Autodesk Fusion 360 part; units mm, degrees
(part 7 of 8)
equation "d1212 = ( BaseX + LeftRun + FaucetGap + ( RightRun + ModuleGap ) / 2 ) + ( ( ( RightRun - ModuleGap ) / 2 ) / 2 - 8 mm )"
equation "d1213 = ( BaseY ) + ( ( Depth ) - Wall - DeckClearance - 4 mm )"
equation "d1216 = DeckThick"
equation "d1220 = ( BaseX + LeftRun + FaucetGap + ( RightRun + ModuleGap ) / 2 ) + ( ( 11 mm ) - FootSize / 2 )"
equation "d1221 = ( BaseY ) + ( ( 11 mm ) - FootSize / 2 )"
equation "d1222 = FootSize"
equation "d1223 = FootSize"
equation "d1224 = FootHeight"
equation "d1226 = FootHeight"
equation "d1228 = ( BaseX + LeftRun + FaucetGap + ( RightRun + ModuleGap ) / 2 ) + ( ( 11 mm ) - PegSize / 2 )"
equation "d1229 = ( BaseY ) + ( ( 11 mm ) - PegSize / 2 )"
equation "d1230 = PegSize"
equation "d1231 = PegSize"
equation "d1232 = PegHeight"
equation "d1236 = ( BaseX + LeftRun + FaucetGap + ( RightRun + ModuleGap ) / 2 ) + ( ( 11 mm ) - FootSize / 2 )"
equation "d1237 = ( BaseY ) + ( ( ( Depth ) - 11 mm ) - FootSize / 2 )"
equation "d1238 = FootSize"
equation "d1239 = FootSize"
equation "d1240 = FootHeight"
equation "d1242 = FootHeight"
equation "d1244 = ( BaseX + LeftRun + FaucetGap + ( RightRun + ModuleGap ) / 2 ) + ( ( 11 mm ) - PegSize / 2 )"
equation "d1245 = ( BaseY ) + ( ( ( Depth ) - 11 mm ) - PegSize / 2 )"
equation "d1246 = PegSize"
equation "d1247 = PegSize"
equation "d1248 = PegHeight"
equation "d1252 = ( BaseX + LeftRun + FaucetGap + ( RightRun + ModuleGap ) / 2 ) + ( ( ( ( RightRun - ModuleGap ) / 2 ) - 11 mm ) - FootSize / 2 )"
equation "d1253 = ( BaseY ) + ( ( 11 mm ) - FootSize / 2 )"
equation "d1254 = FootSize"
equation "d1255 = FootSize"
equation "d1256 = FootHeight"
equation "d1258 = FootHeight"
equation "d1260 = ( BaseX + LeftRun + FaucetGap + ( RightRun + ModuleGap ) / 2 ) + ( ( ( ( RightRun - ModuleGap ) / 2 ) - 11 mm ) - PegSize / 2 )"
equation "d1261 = ( BaseY ) + ( ( 11 mm ) - PegSize / 2 )"
equation "d1262 = PegSize"
equation "d1263 = PegSize"
equation "d1264 = PegHeight"
equation "d1268 = ( BaseX + LeftRun + FaucetGap + ( RightRun + ModuleGap ) / 2 ) + ( ( ( ( RightRun - ModuleGap ) / 2 ) - 11 mm ) - FootSize / 2 )"
equation "d1269 = ( BaseY ) + ( ( ( Depth ) - 11 mm ) - FootSize / 2 )"
equation "d1270 = FootSize"
equation "d1271 = FootSize"
equation "d1272 = FootHeight"
equation "d1274 = FootHeight"
equation "d1276 = ( BaseX + LeftRun + FaucetGap + ( RightRun + ModuleGap ) / 2 ) + ( ( ( ( RightRun - ModuleGap ) / 2 ) - 11 mm ) - PegSize / 2 )"
equation "d1277 = ( BaseY ) + ( ( ( Depth ) - 11 mm ) - PegSize / 2 )"
equation "d1278 = PegSize"
equation "d1279 = PegSize"
equation "d1280 = PegHeight"
equation "d1282 = FootHeight"
equation "d1284 = ( BaseX ) + ( 0 mm )"
equation "d1285 = ( BaseY + Depth + ModuleGap ) + ( ( LeftReach ) - ( ( 0 mm ) + ( LeftReach ) ) )"
equation "d1286 = LeftSideDepth"
equation "d1287 = LeftReach"
equation "d1288 = PanHeight"
equation "d1292 = ( BaseY + Depth + ModuleGap ) + ( ( LeftReach ) - ( Wall ) )"
equation "d1294 = ( ( BaseX ) + ( Wall ) )"
equation "d1295 = -( -( ( FootHeight ) + FloorMin + DrainExtension * tan(DrainSlope) + ( ( LeftSideDepth ) - ( Wall ) ) * tan(DrainSlope) ) )"
equation "d1296 = ( ( BaseX ) + ( ( LeftSideDepth ) - Wall ) )"
equation "d1297 = -( -( ( FootHeight ) + FloorMin + DrainExtension * tan(DrainSlope) + ( ( LeftSideDepth ) - ( ( LeftSideDepth ) - Wall ) ) * tan(DrainSlope) ) )"
equation "d1298 = -( -( ( FootHeight ) + PanHeight + 1 mm ) )"
equation "d1299 = -( -( -( ( LeftReach ) - 2 * Wall ) ) )"
equation "d1301 = ( BaseY + Depth + ModuleGap ) + ( ( LeftReach ) - ( ( LeftReach / 2 ) - DrainWidth / 2 - Wall ) )"
equation "d1303 = ( ( BaseX ) + ( ( LeftSideDepth ) - Wall ) )"
equation "d1304 = -( -( FootHeight ) )"
equation "d1305 = ( ( BaseX ) + ( ( LeftSideDepth ) + DrainExtension ) )"
equation "d1306 = -( -( ( FootHeight ) + FloorMin + DrainExtension * tan(DrainSlope) + ( ( LeftSideDepth ) - ( ( LeftSideDepth ) + DrainExtension ) ) * tan(DrainSlope) ) )"
equation "d1307 = -( -( ( FootHeight ) + FloorMin + DrainExtension * tan(DrainSlope) + ( ( LeftSideDepth ) - ( ( LeftSideDepth ) - Wall ) ) * tan(DrainSlope) ) )"
equation "d1308 = -( DrainWidth + 2 * Wall )"
equation "d1310 = ( BaseY + Depth + ModuleGap ) + ( ( LeftReach ) - ( ( LeftReach / 2 ) - DrainWidth / 2 - Wall ) )"
equation "d1312 = ( ( BaseX ) + ( ( LeftSideDepth ) - Wall ) )"
equation "d1313 = -( -( FootHeight ) )"
equation "d1314 = ( ( BaseX ) + ( ( LeftSideDepth ) + DrainExtension ) )"
equation "d1315 = -( -( ( ( FootHeight ) + FloorMin + DrainExtension * tan(DrainSlope) + ( ( LeftSideDepth ) - ( ( LeftSideDepth ) + DrainExtension ) ) * tan(DrainSlope) ) + ( 6 mm ) ) )"
equation "d1316 = -( -( ( ( FootHeight ) + FloorMin + DrainExtension * tan(DrainSlope) + ( ( LeftSideDepth ) - ( ( LeftSideDepth ) - Wall ) ) * tan(DrainSlope) ) + ( 6 mm ) ) )"
equation "d1317 = -( Wall )"
equation "d1319 = ( BaseY + Depth + ModuleGap ) + ( ( LeftReach ) - ( ( LeftReach / 2 ) + DrainWidth / 2 ) )"
equation "d1321 = ( ( BaseX ) + ( ( LeftSideDepth ) - Wall ) )"
equation "d1322 = -( -( FootHeight ) )"
equation "d1323 = ( ( BaseX ) + ( ( LeftSideDepth ) + DrainExtension ) )"
equation "d1324 = -( -( ( ( FootHeight ) + FloorMin + DrainExtension * tan(DrainSlope) + ( ( LeftSideDepth ) - ( ( LeftSideDepth ) + DrainExtension ) ) * tan(DrainSlope) ) + ( 6 mm ) ) )"
equation "d1325 = -( -( ( ( FootHeight ) + FloorMin + DrainExtension * tan(DrainSlope) + ( ( LeftSideDepth ) - ( ( LeftSideDepth ) - Wall ) ) * tan(DrainSlope) ) + ( 6 mm ) ) )"
equation "d1326 = -( Wall )"
equation "d1328 = ( BaseY + Depth + ModuleGap ) + ( ( LeftReach ) - ( ( LeftReach / 2 ) - DrainWidth / 2 ) )"
equation "d1330 = ( ( BaseX ) + ( ( LeftSideDepth ) - Wall ) )"
equation "d1331 = -( -( ( FootHeight ) + FloorMin + DrainExtension * tan(DrainSlope) + ( ( LeftSideDepth ) - ( ( LeftSideDepth ) - Wall ) ) * tan(DrainSlope) ) )"
equation "d1332 = ( ( BaseX ) + ( ( LeftSideDepth ) + DrainExtension ) )"
equation "d1333 = -( -( ( FootHeight ) + FloorMin + DrainExtension * tan(DrainSlope) + ( ( LeftSideDepth ) - ( ( LeftSideDepth ) + DrainExtension ) ) * tan(DrainSlope) ) )"
equation "d1334 = -( -( ( FootHeight ) + PanHeight + 1 mm ) )"
equation "d1335 = -( -( -( DrainWidth ) ) )"
equation "d1337 = FootHeight"
equation "d1339 = ( BaseX ) + ( Wall )"
equation "d1340 = ( BaseY + Depth + ModuleGap ) + ( ( LeftReach ) - ( ( Wall ) + ( 12 mm ) ) )"
equation "d1343 = PanHeight - DeckThick"
equation "d1345 = FootHeight"
equation "d1347 = ( BaseX ) + ( ( LeftSideDepth ) - Wall - 12 mm )"
equation "d1348 = ( BaseY + Depth + ModuleGap ) + ( ( LeftReach ) - ( ( Wall ) + ( 12 mm ) ) )"
equation "d1351 = PanHeight - DeckThick"
equation "d1353 = FootHeight"
equation "d1355 = ( BaseX ) + ( Wall )"
equation "d1356 = ( BaseY + Depth + ModuleGap ) + ( ( LeftReach ) - ( ( ( LeftReach ) - Wall - 12 mm ) + ( 12 mm ) ) )"
equation "d1359 = PanHeight - DeckThick"
equation "d1361 = FootHeight"
equation "d1363 = ( BaseX ) + ( ( LeftSideDepth ) - Wall - 12 mm )"
equation "d1364 = ( BaseY + Depth + ModuleGap ) + ( ( LeftReach ) - ( ( ( LeftReach ) - Wall - 12 mm ) + ( 12 mm ) ) )"
equation "d1367 = PanHeight - DeckThick"
equation "d1369 = ( BaseY + Depth + ModuleGap ) + ( ( LeftReach ) - ( ( LeftReach / 2 ) - DrainWidth / 2 - Wall ) )"
equation "d1371 = ( ( BaseX ) + ( ( LeftSideDepth ) + DrainExtension - 2 mm ) )"
equation "d1372 = -( -( ( FootHeight ) - ( 0.2 mm ) ) )"
equation "d1373 = ( ( BaseX ) + ( ( ( LeftSideDepth ) + DrainExtension - 2 mm ) + ( 1 mm ) ) )"
equation "d1374 = -( -( ( FootHeight ) + ( 0.6 mm ) ) )"
equation "d1375 = -( -( -( DrainWidth + 2 * Wall ) ) )"
equation "d1377 = FootHeight"
equation "d1379 = ( BaseX ) + ( ( 11 mm ) - PegSize / 2 - FitClearance )"
equation "d1380 = ( BaseY + Depth + ModuleGap ) + ( ( LeftReach ) - ( ( ( 11 mm ) - PegSize / 2 - FitClearance ) + ( PegSize + 2 * FitClearance ) ) )"
equation "d1381 = PegSize + 2 * FitClearance"
equation "d1382 = PegSize + 2 * FitClearance"
equation "d1383 = PegHeight + 0.3 mm"
equation "d1385 = FootHeight"
equation "d1387 = ( BaseX ) + ( ( ( LeftSideDepth ) - 11 mm ) - PegSize / 2 - FitClearance )"
equation "d1388 = ( BaseY + Depth + ModuleGap ) + ( ( LeftReach ) - ( ( ( 11 mm ) - PegSize / 2 - FitClearance ) + ( PegSize + 2 * FitClearance ) ) )"
equation "d1389 = PegSize + 2 * FitClearance"
equation "d1390 = PegSize + 2 * FitClearance"
equation "d1391 = PegHeight + 0.3 mm"
equation "d1393 = FootHeight"
equation "d1395 = ( BaseX ) + ( ( 11 mm ) - PegSize / 2 - FitClearance )"
equation "d1396 = ( BaseY + Depth + ModuleGap ) + ( ( LeftReach ) - ( ( ( ( LeftReach ) - 11 mm ) - PegSize / 2 - FitClearance ) + ( PegSize + 2 * FitClearance ) ) )"
equation "d1397 = PegSize + 2 * FitClearance"
equation "d1398 = PegSize + 2 * FitClearance"
equation "d1399 = PegHeight + 0.3 mm"
equation "d1401 = FootHeight"
equation "d1403 = ( BaseX ) + ( ( ( LeftSideDepth ) - 11 mm ) - PegSize / 2 - FitClearance )"
equation "d1404 = ( BaseY + Depth + ModuleGap ) + ( ( LeftReach ) - ( ( ( ( LeftReach ) - 11 mm ) - PegSize / 2 - FitClearance ) + ( PegSize + 2 * FitClearance ) ) )"
equation "d1405 = PegSize + 2 * FitClearance"
equation "d1406 = PegSize + 2 * FitClearance"
equation "d1407 = PegHeight + 0.3 mm"
equation "d1409 = ( FootHeight ) + PanHeight - DeckThick"
equation "d1411 = ( BaseX ) + ( Wall + DeckClearance )"
equation "d1412 = ( BaseY + Depth + ModuleGap ) + ( ( LeftReach ) - ( ( Wall + DeckClearance ) + ( ( LeftReach ) - 2 * ( Wall + DeckClearance ) ) ) )"
equation "d1413 = ( LeftSideDepth ) - 2 * ( Wall + DeckClearance )"
equation "d1414 = ( LeftReach ) - 2 * ( Wall + DeckClearance )"
equation "d1415 = DeckThick"
equation "d1417 = ( FootHeight ) + PanHeight - DeckThick"
equation "d1419 = ( BaseX ) + ( Wall + DeckClearance + RimBorder )"
equation "d1420 = ( BaseY + Depth + ModuleGap ) + ( ( LeftReach ) - ( ( ( ( ( LeftReach ) - ( 14 * SlotPitch + SlotWidth ) ) / 2 ) + ( 0 * SlotPitch ) ) + ( SlotWidth ) ) )"
equation "d1421 = ( LeftSideDepth ) - 2 * ( Wall + DeckClearance + RimBorder )"
equation "d1422 = SlotWidth"
equation "d1423 = DeckThick"
equation "d1425 = ( FootHeight ) + PanHeight - DeckThick"
equation "d1427 = ( BaseX ) + ( Wall + DeckClearance + RimBorder )"
equation "d1428 = ( BaseY + Depth + ModuleGap ) + ( ( LeftReach ) - ( ( ( ( ( LeftReach ) - ( 14 * SlotPitch + SlotWidth ) ) / 2 ) + ( 1 * SlotPitch ) ) + ( SlotWidth ) ) )"
equation "d1429 = ( LeftSideDepth ) - 2 * ( Wall + DeckClearance + RimBorder )"
equation "d1430 = SlotWidth"
equation "d1431 = DeckThick"
equation "d1433 = ( FootHeight ) + PanHeight - DeckThick"
equation "d1435 = ( BaseX ) + ( Wall + DeckClearance + RimBorder )"
equation "d1436 = ( BaseY + Depth + ModuleGap ) + ( ( LeftReach ) - ( ( ( ( ( LeftReach ) - ( 14 * SlotPitch + SlotWidth ) ) / 2 ) + ( 2 * SlotPitch ) ) + ( SlotWidth ) ) )"
equation "d1437 = ( LeftSideDepth ) - 2 * ( Wall + DeckClearance + RimBorder )"
equation "d1438 = SlotWidth"
equation "d1439 = DeckThick"
equation "d1441 = ( FootHeight ) + PanHeight - DeckThick"
equation "d1443 = ( BaseX ) + ( Wall + DeckClearance + RimBorder )"
equation "d1444 = ( BaseY + Depth + ModuleGap ) + ( ( LeftReach ) - ( ( ( ( ( LeftReach ) - ( 14 * SlotPitch + SlotWidth ) ) / 2 ) + ( 3 * SlotPitch ) ) + ( SlotWidth ) ) )"
equation "d1445 = ( LeftSideDepth ) - 2 * ( Wall + DeckClearance + RimBorder )"
equation "d1446 = SlotWidth"
equation "d1447 = DeckThick"
equation "d1449 = ( FootHeight ) + PanHeight - DeckThick"
equation "d1451 = ( BaseX ) + ( Wall + DeckClearance + RimBorder )"
equation "d1452 = ( BaseY + Depth + ModuleGap ) + ( ( LeftReach ) - ( ( ( ( ( LeftReach ) - ( 14 * SlotPitch + SlotWidth ) ) / 2 ) + ( 4 * SlotPitch ) ) + ( SlotWidth ) ) )"
equation "d1453 = ( LeftSideDepth ) - 2 * ( Wall + DeckClearance + RimBorder )"
equation "d1454 = SlotWidth"
equation "d1455 = DeckThick"
equation "d1457 = ( FootHeight ) + PanHeight - DeckThick"
equation "d1459 = ( BaseX ) + ( Wall + DeckClearance + RimBorder )"
equation "d1460 = ( BaseY + Depth + ModuleGap ) + ( ( LeftReach ) - ( ( ( ( ( LeftReach ) - ( 14 * SlotPitch + SlotWidth ) ) / 2 ) + ( 5 * SlotPitch ) ) + ( SlotWidth ) ) )"
equation "d1461 = ( LeftSideDepth ) - 2 * ( Wall + DeckClearance + RimBorder )"
equation "d1462 = SlotWidth"
equation "d1463 = DeckThick"
equation "d1465 = ( FootHeight ) + PanHeight - DeckThick"
equation "d1467 = ( BaseX ) + ( Wall + DeckClearance + RimBorder )"
equation "d1468 = ( BaseY + Depth + ModuleGap ) + ( ( LeftReach ) - ( ( ( ( ( LeftReach ) - ( 14 * SlotPitch + SlotWidth ) ) / 2 ) + ( 6 * SlotPitch ) ) + ( SlotWidth ) ) )"
equation "d1469 = ( LeftSideDepth ) - 2 * ( Wall + DeckClearance + RimBorder )"
equation "d1470 = SlotWidth"
equation "d1471 = DeckThick"
equation "d1473 = ( FootHeight ) + PanHeight - DeckThick"
equation "d1475 = ( BaseX ) + ( Wall + DeckClearance + RimBorder )"
equation "d1476 = ( BaseY + Depth + ModuleGap ) + ( ( LeftReach ) - ( ( ( ( ( LeftReach ) - ( 14 * SlotPitch + SlotWidth ) ) / 2 ) + ( 7 * SlotPitch ) ) + ( SlotWidth ) ) )"
equation "d1477 = ( LeftSideDepth ) - 2 * ( Wall + DeckClearance + RimBorder )"
equation "d1478 = SlotWidth"
equation "d1479 = DeckThick"
equation "d1481 = ( FootHeight ) + PanHeight - DeckThick"
equation "d1483 = ( BaseX ) + ( Wall + DeckClearance + RimBorder )"
equation "d1484 = ( BaseY + Depth + ModuleGap ) + ( ( LeftReach ) - ( ( ( ( ( LeftReach ) - ( 14 * SlotPitch + SlotWidth ) ) / 2 ) + ( 8 * SlotPitch ) ) + ( SlotWidth ) ) )"
equation "d1485 = ( LeftSideDepth ) - 2 * ( Wall + DeckClearance + RimBorder )"
equation "d1486 = SlotWidth"
equation "d1487 = DeckThick"
equation "d1489 = ( FootHeight ) + PanHeight - DeckThick"
equation "d1491 = ( BaseX ) + ( Wall + DeckClearance + RimBorder )"
equation "d1492 = ( BaseY + Depth + ModuleGap ) + ( ( LeftReach ) - ( ( ( ( ( LeftReach ) - ( 14 * SlotPitch + SlotWidth ) ) / 2 ) + ( 9 * SlotPitch ) ) + ( SlotWidth ) ) )"
equation "d1493 = ( LeftSideDepth ) - 2 * ( Wall + DeckClearance + RimBorder )"
equation "d1494 = SlotWidth"
equation "d1495 = DeckThick"
equation "d1497 = ( FootHeight ) + PanHeight - DeckThick"
equation "d1499 = ( BaseX ) + ( Wall + DeckClearance + RimBorder )"
equation "d1500 = ( BaseY + Depth + ModuleGap ) + ( ( LeftReach ) - ( ( ( ( ( LeftReach ) - ( 14 * SlotPitch + SlotWidth ) ) / 2 ) + ( 10 * SlotPitch ) ) + ( SlotWidth ) ) )"
equation "d1501 = ( LeftSideDepth ) - 2 * ( Wall + DeckClearance + RimBorder )"
equation "d1502 = SlotWidth"
equation "d1503 = DeckThick"
equation "d1505 = ( FootHeight ) + PanHeight - DeckThick"
equation "d1507 = ( BaseX ) + ( Wall + DeckClearance + RimBorder )"
equation "d1508 = ( BaseY + Depth + ModuleGap ) + ( ( LeftReach ) - ( ( ( ( ( LeftReach ) - ( 14 * SlotPitch + SlotWidth ) ) / 2 ) + ( 11 * SlotPitch ) ) + ( SlotWidth ) ) )"
equation "d1509 = ( LeftSideDepth ) - 2 * ( Wall + DeckClearance + RimBorder )"
equation "d1510 = SlotWidth"
equation "d1511 = DeckThick"
equation "d1513 = ( FootHeight ) + PanHeight - DeckThick"
equation "d1515 = ( BaseX ) + ( Wall + DeckClearance + RimBorder )"
equation "d1516 = ( BaseY + Depth + ModuleGap ) + ( ( LeftReach ) - ( ( ( ( ( LeftReach ) - ( 14 * SlotPitch + SlotWidth ) ) / 2 ) + ( 12 * SlotPitch ) ) + ( SlotWidth ) ) )"
equation "d1517 = ( LeftSideDepth ) - 2 * ( Wall + DeckClearance + RimBorder )"
equation "d1518 = SlotWidth"
equation "d1519 = DeckThick"
equation "d1521 = ( FootHeight ) + PanHeight - DeckThick"
equation "d1523 = ( BaseX ) + ( Wall + DeckClearance + RimBorder )"
equation "d1524 = ( BaseY + Depth + ModuleGap ) + ( ( LeftReach ) - ( ( ( ( ( LeftReach ) - ( 14 * SlotPitch + SlotWidth ) ) / 2 ) + ( 13 * SlotPitch ) ) + ( SlotWidth ) ) )"
equation "d1525 = ( LeftSideDepth ) - 2 * ( Wall + DeckClearance + RimBorder )"
equation "d1526 = SlotWidth"
equation "d1527 = DeckThick"
equation "d1529 = ( FootHeight ) + PanHeight - DeckThick"
equation "d1531 = ( BaseX ) + ( Wall + DeckClearance + RimBorder )"
equation "d1532 = ( BaseY + Depth + ModuleGap ) + ( ( LeftReach ) - ( ( ( ( ( LeftReach ) - ( 14 * SlotPitch + SlotWidth ) ) / 2 ) + ( 14 * SlotPitch ) ) + ( SlotWidth ) ) )"
equation "d1533 = ( LeftSideDepth ) - 2 * ( Wall + DeckClearance + RimBorder )"
equation "d1534 = SlotWidth"
equation "d1535 = DeckThick"
equation "d1537 = ( FootHeight ) + PanHeight - DeckThick"
equation "d1539 = ( BaseX ) + ( ( LeftSideDepth ) - Wall - DeckClearance - 4 mm )"
equation "d1540 = ( BaseY + Depth + ModuleGap ) + ( ( LeftReach ) - ( ( ( LeftReach ) / 2 - 8 mm ) + ( 16 mm ) ) )"
equation "d1543 = DeckThick"
equation "d1547 = ( BaseX ) + ( ( 11 mm ) - FootSize / 2 )"
equation "d1548 = ( BaseY + Depth + ModuleGap ) + ( ( LeftReach ) - ( ( ( 11 mm ) - FootSize / 2 ) + ( FootSize ) ) )"
equation "d1549 = FootSize"
equation "d1550 = FootSize"
equation "d1551 = FootHeight"
equation "d1553 = FootHeight"
equation "d1555 = ( BaseX ) + ( ( 11 mm ) - PegSize / 2 )"
equation "d1556 = ( BaseY + Depth + ModuleGap ) + ( ( LeftReach ) - ( ( ( 11 mm ) - PegSize / 2 ) + ( PegSize ) ) )"
equation "d1557 = PegSize"
equation "d1558 = PegSize"
equation "d1559 = PegHeight"
equation "d1563 = ( BaseX ) + ( ( ( LeftSideDepth ) - 11 mm ) - FootSize / 2 )"
equation "d1564 = ( BaseY + Depth + ModuleGap ) + ( ( LeftReach ) - ( ( ( 11 mm ) - FootSize / 2 ) + ( FootSize ) ) )"
equation "d1565 = FootSize"
equation "d1566 = FootSize"
equation "d1567 = FootHeight"
equation "d1569 = FootHeight"
equation "d1571 = ( BaseX ) + ( ( ( LeftSideDepth ) - 11 mm ) - PegSize / 2 )"
equation "d1572 = ( BaseY + Depth + ModuleGap ) + ( ( LeftReach ) - ( ( ( 11 mm ) - PegSize / 2 ) + ( PegSize ) ) )"
equation "d1573 = PegSize"
equation "d1574 = PegSize"
equation "d1575 = PegHeight"
equation "d1579 = ( BaseX ) + ( ( 11 mm ) - FootSize / 2 )"
equation "d1580 = ( BaseY + Depth + ModuleGap ) + ( ( LeftReach ) - ( ( ( ( LeftReach ) - 11 mm ) - FootSize / 2 ) + ( FootSize ) ) )"
equation "d1581 = FootSize"
equation "d1582 = FootSize"
equation "d1583 = FootHeight"
equation "d1585 = FootHeight"
equation "d1587 = ( BaseX ) + ( ( 11 mm ) - PegSize / 2 )"
equation "d1588 = ( BaseY + Depth + ModuleGap ) + ( ( LeftReach ) - ( ( ( ( LeftReach ) - 11 mm ) - PegSize / 2 ) + ( PegSize ) ) )"
equation "d1589 = PegSize"
equation "d1590 = PegSize"
equation "d1591 = PegHeight"
equation "d1595 = ( BaseX ) + ( ( ( LeftSideDepth ) - 11 mm ) - FootSize / 2 )"
equation "d1596 = ( BaseY + Depth + ModuleGap ) + ( ( LeftReach ) - ( ( ( ( LeftReach ) - 11 mm ) - FootSize / 2 ) + ( FootSize ) ) )"
equation "d1597 = FootSize"
equation "d1598 = FootSize"
equation "d1599 = FootHeight"
equation "d1601 = FootHeight"
equation "d1603 = ( BaseX ) + ( ( ( LeftSideDepth ) - 11 mm ) - PegSize / 2 )"
equation "d1604 = ( BaseY + Depth + ModuleGap ) + ( ( LeftReach ) - ( ( ( ( LeftReach ) - 11 mm ) - PegSize / 2 ) + ( PegSize ) ) )"
equation "d1605 = PegSize"
equation "d1606 = PegSize"
equation "d1607 = PegHeight"
equation "d1609 = FootHeight"
equation "d1611 = ( BaseX + LeftRun + FaucetGap + RightRun - RightSideDepth ) + ( ( RightSideDepth ) - ( ( 0 mm ) + ( RightSideDepth ) ) )"
equation "d1612 = ( BaseY + Depth + ModuleGap ) + ( 0 mm )"
equation "d1613 = RightSideDepth"
equation "d1614 = RightReach"
equation "d1615 = PanHeight"
equation "d1619 = ( BaseY + Depth + ModuleGap ) + ( Wall )"
equation "d1621 = ( ( BaseX + LeftRun + FaucetGap + RightRun - RightSideDepth ) + ( ( RightSideDepth ) - ( Wall ) ) )"
equation "d1622 = -( -( ( FootHeight ) + FloorMin + DrainExtension * tan(DrainSlope) + ( ( RightSideDepth ) - ( Wall ) ) * tan(DrainSlope) ) )"
equation "d1623 = ( ( BaseX + LeftRun + FaucetGap + RightRun - RightSideDepth ) + ( ( RightSideDepth ) - ( ( RightSideDepth ) - Wall ) ) )"
equation "d1624 = -( -( ( FootHeight ) + FloorMin + DrainExtension * tan(DrainSlope) + ( ( RightSideDepth ) - ( ( RightSideDepth ) - Wall ) ) * tan(DrainSlope) ) )"
equation "d1625 = -( -( ( FootHeight ) + PanHeight + 1 mm ) )"
equation "d1626 = ( RightReach ) - 2 * Wall"
equation "d1628 = ( BaseY + Depth + ModuleGap ) + ( ( RightReach / 2 ) - DrainWidth / 2 - Wall )"
equation "d1630 = ( ( BaseX + LeftRun + FaucetGap + RightRun - RightSideDepth ) + ( ( RightSideDepth ) - ( ( RightSideDepth ) - Wall ) ) )"
equation "d1631 = -( -( FootHeight ) )"
equation "d1632 = ( ( BaseX + LeftRun + FaucetGap + RightRun - RightSideDepth ) + ( ( RightSideDepth ) - ( ( RightSideDepth ) + DrainExtension ) ) )"
equation "d1633 = -( -( ( FootHeight ) + FloorMin + DrainExtension * tan(DrainSlope) + ( ( RightSideDepth ) - ( ( RightSideDepth ) + DrainExtension ) ) * tan(DrainSlope) ) )"
equation "d1634 = -( -( ( FootHeight ) + FloorMin + DrainExtension * tan(DrainSlope) + ( ( RightSideDepth ) - ( ( RightSideDepth ) - Wall ) ) * tan(DrainSlope) ) )"
equation "d1635 = DrainWidth + 2 * Wall"
equation "d1637 = ( BaseY + Depth + ModuleGap ) + ( ( RightReach / 2 ) - DrainWidth / 2 - Wall )"
equation "d1639 = ( ( BaseX + LeftRun + FaucetGap + RightRun - RightSideDepth ) + ( ( RightSideDepth ) - ( ( RightSideDepth ) - Wall ) ) )"
equation "d1640 = -( -( FootHeight ) )"
equation "d1641 = ( ( BaseX + LeftRun + FaucetGap + RightRun - RightSideDepth ) + ( ( RightSideDepth ) - ( ( RightSideDepth ) + DrainExtension ) ) )"
equation "d1642 = -( -( ( ( FootHeight ) + FloorMin + DrainExtension * tan(DrainSlope) + ( ( RightSideDepth ) - ( ( RightSideDepth ) + DrainExtension ) ) * tan(DrainSlope) ) + ( 6 mm ) ) )"
equation "d1643 = -( -( ( ( FootHeight ) + FloorMin + DrainExtension * tan(DrainSlope) + ( ( RightSideDepth ) - ( ( RightSideDepth ) - Wall ) ) * tan(DrainSlope) ) + ( 6 mm ) ) )"
equation "d1644 = Wall"
equation "d1646 = ( BaseY + Depth + ModuleGap ) + ( ( RightReach / 2 ) + DrainWidth / 2 )"
equation "d1648 = ( ( BaseX + LeftRun + FaucetGap + RightRun - RightSideDepth ) + ( ( RightSideDepth ) - ( ( RightSideDepth ) - Wall ) ) )"
equation "d1649 = -( -( FootHeight ) )"
equation "d1650 = ( ( BaseX + LeftRun + FaucetGap + RightRun - RightSideDepth ) + ( ( RightSideDepth ) - ( ( RightSideDepth ) + DrainExtension ) ) )"
equation "d1651 = -( -( ( ( FootHeight ) + FloorMin + DrainExtension * tan(DrainSlope) + ( ( RightSideDepth ) - ( ( RightSideDepth ) + DrainExtension ) ) * tan(DrainSlope) ) + ( 6 mm ) ) )"
equation "d1652 = -( -( ( ( FootHeight ) + FloorMin + DrainExtension * tan(DrainSlope) + ( ( RightSideDepth ) - ( ( RightSideDepth ) - Wall ) ) * tan(DrainSlope) ) + ( 6 mm ) ) )"
equation "d1653 = Wall"
equation "d1655 = ( BaseY + Depth + ModuleGap ) + ( ( RightReach / 2 ) - DrainWidth / 2 )"
equation "d1657 = ( ( BaseX + LeftRun + FaucetGap + RightRun - RightSideDepth ) + ( ( RightSideDepth ) - ( ( RightSideDepth ) - Wall ) ) )"
equation "d1658 = -( -( ( FootHeight ) + FloorMin + DrainExtension * tan(DrainSlope) + ( ( RightSideDepth ) - ( ( RightSideDepth ) - Wall ) ) * tan(DrainSlope) ) )"
equation "d1659 = ( ( BaseX + LeftRun + FaucetGap + RightRun - RightSideDepth ) + ( ( RightSideDepth ) - ( ( RightSideDepth ) + DrainExtension ) ) )"
equation "d1660 = -( -( ( FootHeight ) + FloorMin + DrainExtension * tan(DrainSlope) + ( ( RightSideDepth ) - ( ( RightSideDepth ) + DrainExtension ) ) * tan(DrainSlope) ) )"
equation "d1661 = -( -( ( FootHeight ) + PanHeight + 1 mm ) )"
equation "d1662 = DrainWidth"
equation "d1664 = FootHeight"
equation "d1666 = ( BaseX + LeftRun + FaucetGap + RightRun - RightSideDepth ) + ( ( RightSideDepth ) - ( ( Wall ) + ( 12 mm ) ) )"
equation "d1667 = ( BaseY + Depth + ModuleGap ) + ( Wall )"
equation "d1670 = PanHeight - DeckThick"
equation "d1672 = FootHeight"
equation "d1674 = ( BaseX + LeftRun + FaucetGap + RightRun - RightSideDepth ) + ( ( RightSideDepth ) - ( ( ( RightSideDepth ) - Wall - 12 mm ) + ( 12 mm ) ) )"
equation "d1675 = ( BaseY + Depth + ModuleGap ) + ( Wall )"
equation "d1678 = PanHeight - DeckThick"
equation "d1680 = FootHeight"
equation "d1682 = ( BaseX + LeftRun + FaucetGap + RightRun - RightSideDepth ) + ( ( RightSideDepth ) - ( ( Wall ) + ( 12 mm ) ) )"
equation "d1683 = ( BaseY + Depth + ModuleGap ) + ( ( RightReach ) - Wall - 12 mm )"
equation "d1686 = PanHeight - DeckThick"
equation "d1688 = FootHeight"
equation "d1690 = ( BaseX + LeftRun + FaucetGap + RightRun - RightSideDepth ) + ( ( RightSideDepth ) - ( ( ( RightSideDepth ) - Wall - 12 mm ) + ( 12 mm ) ) )"
equation "d1691 = ( BaseY + Depth + ModuleGap ) + ( ( RightReach ) - Wall - 12 mm )"
equation "d1694 = PanHeight - DeckThick"
equation "d1696 = ( BaseY + Depth + ModuleGap ) + ( ( RightReach / 2 ) - DrainWidth / 2 - Wall )"
equation "d1698 = ( ( BaseX + LeftRun + FaucetGap + RightRun - RightSideDepth ) + ( ( RightSideDepth ) - ( ( RightSideDepth ) + DrainExtension - 2 mm ) ) )"
equation "d1699 = -( -( ( FootHeight ) - ( 0.2 mm ) ) )"
equation "d1700 = ( ( BaseX + LeftRun + FaucetGap + RightRun - RightSideDepth ) + ( ( RightSideDepth ) - ( ( ( RightSideDepth ) + DrainExtension - 2 mm ) + ( 1 mm ) ) ) )"
equation "d1701 = -( -( ( FootHeight ) + ( 0.6 mm ) ) )"
equation "d1702 = DrainWidth + 2 * Wall"
equation "d1704 = FootHeight"
equation "d1706 = ( BaseX + LeftRun + FaucetGap + RightRun - RightSideDepth ) + ( ( RightSideDepth ) - ( ( ( 11 mm ) - PegSize / 2 - FitClearance ) + ( PegSize + 2 * FitClearance ) ) )"
equation "d1707 = ( BaseY + Depth + ModuleGap ) + ( ( 11 mm ) - PegSize / 2 - FitClearance )"
equation "d1708 = PegSize + 2 * FitClearance"
equation "d1709 = PegSize + 2 * FitClearance"
equation "d1710 = PegHeight + 0.3 mm"
equation "d1712 = FootHeight"
equation "d1714 = ( BaseX + LeftRun + FaucetGap + RightRun - RightSideDepth ) + ( ( RightSideDepth ) - ( ( ( ( RightSideDepth ) - 11 mm ) - PegSize / 2 - FitClearance ) + ( PegSize + 2 * FitClearance ) ) )"
equation "d1715 = ( BaseY + Depth + ModuleGap ) + ( ( 11 mm ) - PegSize / 2 - FitClearance )"
equation "d1716 = PegSize + 2 * FitClearance"
equation "d1717 = PegSize + 2 * FitClearance"
equation "d1718 = PegHeight + 0.3 mm"
equation "d1720 = FootHeight"
equation "d1722 = ( BaseX + LeftRun + FaucetGap + RightRun - RightSideDepth ) + ( ( RightSideDepth ) - ( ( ( 11 mm ) - PegSize / 2 - FitClearance ) + ( PegSize + 2 * FitClearance ) ) )"
equation "d1723 = ( BaseY + Depth + ModuleGap ) + ( ( ( RightReach ) - 11 mm ) - PegSize / 2 - FitClearance )"
equation "d1724 = PegSize + 2 * FitClearance"
equation "d1725 = PegSize + 2 * FitClearance"
equation "d1726 = PegHeight + 0.3 mm"
equation "d1728 = FootHeight"
equation "d1730 = ( BaseX + LeftRun + FaucetGap + RightRun - RightSideDepth ) + ( ( RightSideDepth ) - ( ( ( ( RightSideDepth ) - 11 mm ) - PegSize / 2 - FitClearance ) + ( PegSize + 2 * FitClearance ) ) )"
equation "d1731 = ( BaseY + Depth + ModuleGap ) + ( ( ( RightReach ) - 11 mm ) - PegSize / 2 - FitClearance )"
equation "d1732 = PegSize + 2 * FitClearance"
equation "d1733 = PegSize + 2 * FitClearance"
equation "d1734 = PegHeight + 0.3 mm"
equation "d1736 = ( FootHeight ) + PanHeight - DeckThick"
equation "d1738 = ( BaseX + LeftRun + FaucetGap + RightRun - RightSideDepth ) + ( ( RightSideDepth ) - ( ( Wall + DeckClearance ) + ( ( RightSideDepth ) - 2 * ( Wall + DeckClearance ) ) ) )"
equation "d1739 = ( BaseY + Depth + ModuleGap ) + ( Wall + DeckClearance )"
equation "d1740 = ( RightSideDepth ) - 2 * ( Wall + DeckClearance )"
equation "d1741 = ( RightReach ) - 2 * ( Wall + DeckClearance )"
equation "d1742 = DeckThick"
equation "d1744 = ( FootHeight ) + PanHeight - DeckThick"
equation "d1746 = ( BaseX + LeftRun + FaucetGap + RightRun - RightSideDepth ) + ( ( RightSideDepth ) - ( ( Wall + DeckClearance + RimBorder ) + ( ( RightSideDepth ) - 2 * ( Wall + DeckClearance + RimBorder ) ) ) )"
equation "d1747 = ( BaseY + Depth + ModuleGap ) + ( ( ( ( RightReach ) - ( 14 * SlotPitch + SlotWidth ) ) / 2 ) + ( 0 * SlotPitch ) )"
equation "d1748 = ( RightSideDepth ) - 2 * ( Wall + DeckClearance + RimBorder )"
equation "d1749 = SlotWidth"
equation "d1750 = DeckThick"
equation "d1752 = ( FootHeight ) + PanHeight - DeckThick"
equation "d1754 = ( BaseX + LeftRun + FaucetGap + RightRun - RightSideDepth ) + ( ( RightSideDepth ) - ( ( Wall + DeckClearance + RimBorder ) + ( ( RightSideDepth ) - 2 * ( Wall + DeckClearance + RimBorder ) ) ) )"
equation "d1755 = ( BaseY + Depth + ModuleGap ) + ( ( ( ( RightReach ) - ( 14 * SlotPitch + SlotWidth ) ) / 2 ) + ( 1 * SlotPitch ) )"
equation "d1756 = ( RightSideDepth ) - 2 * ( Wall + DeckClearance + RimBorder )"
equation "d1757 = SlotWidth"
equation "d1758 = DeckThick"
equation "d1760 = ( FootHeight ) + PanHeight - DeckThick"
equation "d1762 = ( BaseX + LeftRun + FaucetGap + RightRun - RightSideDepth ) + ( ( RightSideDepth ) - ( ( Wall + DeckClearance + RimBorder ) + ( ( RightSideDepth ) - 2 * ( Wall + DeckClearance + RimBorder ) ) ) )"
equation "d1763 = ( BaseY + Depth + ModuleGap ) + ( ( ( ( RightReach ) - ( 14 * SlotPitch + SlotWidth ) ) / 2 ) + ( 2 * SlotPitch ) )"
equation "d1764 = ( RightSideDepth ) - 2 * ( Wall + DeckClearance + RimBorder )"
equation "d1765 = SlotWidth"
equation "d1766 = DeckThick"
equation "d1768 = ( FootHeight ) + PanHeight - DeckThick"
equation "d1770 = ( BaseX + LeftRun + FaucetGap + RightRun - RightSideDepth ) + ( ( RightSideDepth ) - ( ( Wall + DeckClearance + RimBorder ) + ( ( RightSideDepth ) - 2 * ( Wall + DeckClearance + RimBorder ) ) ) )"
equation "d1771 = ( BaseY + Depth + ModuleGap ) + ( ( ( ( RightReach ) - ( 14 * SlotPitch + SlotWidth ) ) / 2 ) + ( 3 * SlotPitch ) )"
equation "d1772 = ( RightSideDepth ) - 2 * ( Wall + DeckClearance + RimBorder )"
equation "d1773 = SlotWidth"
equation "d1774 = DeckThick"
equation "d1776 = ( FootHeight ) + PanHeight - DeckThick"
equation "d1778 = ( BaseX + LeftRun + FaucetGap + RightRun - RightSideDepth ) + ( ( RightSideDepth ) - ( ( Wall + DeckClearance + RimBorder ) + ( ( RightSideDepth ) - 2 * ( Wall + DeckClearance + RimBorder ) ) ) )"
equation "d1779 = ( BaseY + Depth + ModuleGap ) + ( ( ( ( RightReach ) - ( 14 * SlotPitch + SlotWidth ) ) / 2 ) + ( 4 * SlotPitch ) )"
equation "d1780 = ( RightSideDepth ) - 2 * ( Wall + DeckClearance + RimBorder )"
equation "d1781 = SlotWidth"
equation "d1782 = DeckThick"
equation "d1784 = ( FootHeight ) + PanHeight - DeckThick"
equation "d1786 = ( BaseX + LeftRun + FaucetGap + RightRun - RightSideDepth ) + ( ( RightSideDepth ) - ( ( Wall + DeckClearance + RimBorder ) + ( ( RightSideDepth ) - 2 * ( Wall + DeckClearance + RimBorder ) ) ) )"
equation "d1787 = ( BaseY + Depth + ModuleGap ) + ( ( ( ( RightReach ) - ( 14 * SlotPitch + SlotWidth ) ) / 2 ) + ( 5 * SlotPitch ) )"
equation "d1788 = ( RightSideDepth ) - 2 * ( Wall + DeckClearance + RimBorder )"
equation "d1789 = SlotWidth"
equation "d1790 = DeckThick"
equation "d1792 = ( FootHeight ) + PanHeight - DeckThick"
equation "d1794 = ( BaseX + LeftRun + FaucetGap + RightRun - RightSideDepth ) + ( ( RightSideDepth ) - ( ( Wall + DeckClearance + RimBorder ) + ( ( RightSideDepth ) - 2 * ( Wall + DeckClearance + RimBorder ) ) ) )"
equation "d1795 = ( BaseY + Depth + ModuleGap ) + ( ( ( ( RightReach ) - ( 14 * SlotPitch + SlotWidth ) ) / 2 ) + ( 6 * SlotPitch ) )"
equation "d1796 = ( RightSideDepth ) - 2 * ( Wall + DeckClearance + RimBorder )"
equation "d1797 = SlotWidth"
equation "d1798 = DeckThick"
equation "d1800 = ( FootHeight ) + PanHeight - DeckThick"
equation "d1802 = ( BaseX + LeftRun + FaucetGap + RightRun - RightSideDepth ) + ( ( RightSideDepth ) - ( ( Wall + DeckClearance + RimBorder ) + ( ( RightSideDepth ) - 2 * ( Wall + DeckClearance + RimBorder ) ) ) )"
equation "d1803 = ( BaseY + Depth + ModuleGap ) + ( ( ( ( RightReach ) - ( 14 * SlotPitch + SlotWidth ) ) / 2 ) + ( 7 * SlotPitch ) )"
equation "d1804 = ( RightSideDepth ) - 2 * ( Wall + DeckClearance + RimBorder )"
equation "d1805 = SlotWidth"
equation "d1806 = DeckThick"
equation "d1808 = ( FootHeight ) + PanHeight - DeckThick"
equation "d1810 = ( BaseX + LeftRun + FaucetGap + RightRun - RightSideDepth ) + ( ( RightSideDepth ) - ( ( Wall + DeckClearance + RimBorder ) + ( ( RightSideDepth ) - 2 * ( Wall + DeckClearance + RimBorder ) ) ) )"
equation "d1811 = ( BaseY + Depth + ModuleGap ) + ( ( ( ( RightReach ) - ( 14 * SlotPitch + SlotWidth ) ) / 2 ) + ( 8 * SlotPitch ) )"
equation "d1812 = ( RightSideDepth ) - 2 * ( Wall + DeckClearance + RimBorder )"
equation "d1813 = SlotWidth"
equation "d1814 = DeckThick"
equation "d1816 = ( FootHeight ) + PanHeight - DeckThick"
equation "d1818 = ( BaseX + LeftRun + FaucetGap + RightRun - RightSideDepth ) + ( ( RightSideDepth ) - ( ( Wall + DeckClearance + RimBorder ) + ( ( RightSideDepth ) - 2 * ( Wall + DeckClearance + RimBorder ) ) ) )"
equation "d1819 = ( BaseY + Depth + ModuleGap ) + ( ( ( ( RightReach ) - ( 14 * SlotPitch + SlotWidth ) ) / 2 ) + ( 9 * SlotPitch ) )"
equation "d1820 = ( RightSideDepth ) - 2 * ( Wall + DeckClearance + RimBorder )"
equation "d1821 = SlotWidth"
equation "d1822 = DeckThick"
equation "d1824 = ( FootHeight ) + PanHeight - DeckThick"
equation "d1826 = ( BaseX + LeftRun + FaucetGap + RightRun - RightSideDepth ) + ( ( RightSideDepth ) - ( ( Wall + DeckClearance + RimBorder ) + ( ( RightSideDepth ) - 2 * ( Wall + DeckClearance + RimBorder ) ) ) )"
equation "d1827 = ( BaseY + Depth + ModuleGap ) + ( ( ( ( RightReach ) - ( 14 * SlotPitch + SlotWidth ) ) / 2 ) + ( 10 * SlotPitch ) )"
equation "d1828 = ( RightSideDepth ) - 2 * ( Wall + DeckClearance + RimBorder )"
equation "d1829 = SlotWidth"
equation "d1830 = DeckThick"
equation "d1832 = ( FootHeight ) + PanHeight - DeckThick"
equation "d1834 = ( BaseX + LeftRun + FaucetGap + RightRun - RightSideDepth ) + ( ( RightSideDepth ) - ( ( Wall + DeckClearance + RimBorder ) + ( ( RightSideDepth ) - 2 * ( Wall + DeckClearance + RimBorder ) ) ) )"
equation "d1835 = ( BaseY + Depth + ModuleGap ) + ( ( ( ( RightReach ) - ( 14 * SlotPitch + SlotWidth ) ) / 2 ) + ( 11 * SlotPitch ) )"
equation "d1836 = ( RightSideDepth ) - 2 * ( Wall + DeckClearance + RimBorder )"
equation "d1837 = SlotWidth"
equation "d1838 = DeckThick"
equation "d1840 = ( FootHeight ) + PanHeight - DeckThick"
equation "d1842 = ( BaseX + LeftRun + FaucetGap + RightRun - RightSideDepth ) + ( ( RightSideDepth ) - ( ( Wall + DeckClearance + RimBorder ) + ( ( RightSideDepth ) - 2 * ( Wall + DeckClearance + RimBorder ) ) ) )"
equation "d1843 = ( BaseY + Depth + ModuleGap ) + ( ( ( ( RightReach ) - ( 14 * SlotPitch + SlotWidth ) ) / 2 ) + ( 12 * SlotPitch ) )"
equation "d1844 = ( RightSideDepth ) - 2 * ( Wall + DeckClearance + RimBorder )"
equation "d1845 = SlotWidth"
equation "d1846 = DeckThick"
equation "d1848 = ( FootHeight ) + PanHeight - DeckThick"
equation "d1850 = ( BaseX + LeftRun + FaucetGap + RightRun - RightSideDepth ) + ( ( RightSideDepth ) - ( ( Wall + DeckClearance + RimBorder ) + ( ( RightSideDepth ) - 2 * ( Wall + DeckClearance + RimBorder ) ) ) )"
equation "d1851 = ( BaseY + Depth + ModuleGap ) + ( ( ( ( RightReach ) - ( 14 * SlotPitch + SlotWidth ) ) / 2 ) + ( 13 * SlotPitch ) )"
equation "d1852 = ( RightSideDepth ) - 2 * ( Wall + DeckClearance + RimBorder )"
equation "d1853 = SlotWidth"
equation "d1854 = DeckThick"
equation "d1856 = ( FootHeight ) + PanHeight - DeckThick"
equation "d1858 = ( BaseX + LeftRun + FaucetGap + RightRun - RightSideDepth ) + ( ( RightSideDepth ) - ( ( Wall + DeckClearance + RimBorder ) + ( ( RightSideDepth ) - 2 * ( Wall + DeckClearance + RimBorder ) ) ) )"
equation "d1859 = ( BaseY + Depth + ModuleGap ) + ( ( ( ( RightReach ) - ( 14 * SlotPitch + SlotWidth ) ) / 2 ) + ( 14 * SlotPitch ) )"
equation "d1860 = ( RightSideDepth ) - 2 * ( Wall + DeckClearance + RimBorder )"
equation "d1861 = SlotWidth"
equation "d1862 = DeckThick"
equation "d1864 = ( FootHeight ) + PanHeight - DeckThick"
equation "d1866 = ( BaseX + LeftRun + FaucetGap + RightRun - RightSideDepth ) + ( ( RightSideDepth ) - ( ( ( RightSideDepth ) - Wall - DeckClearance - 4 mm ) + ( 5 mm ) ) )"
equation "d1867 = ( BaseY + Depth + ModuleGap ) + ( ( RightReach ) / 2 - 8 mm )"
equation "d1870 = DeckThick"
equation "d1874 = ( BaseX + LeftRun + FaucetGap + RightRun - RightSideDepth ) + ( ( RightSideDepth ) - ( ( ( 11 mm ) - FootSize / 2 ) + ( FootSize ) ) )"
equation "d1875 = ( BaseY + Depth + ModuleGap ) + ( ( 11 mm ) - FootSize / 2 )"
equation "d1876 = FootSize"
equation "d1877 = FootSize"
equation "d1878 = FootHeight"
equation "d1880 = FootHeight"
equation "d1882 = ( BaseX + LeftRun + FaucetGap + RightRun - RightSideDepth ) + ( ( RightSideDepth ) - ( ( ( 11 mm ) - PegSize / 2 ) + ( PegSize ) ) )"
equation "d1883 = ( BaseY + Depth + ModuleGap ) + ( ( 11 mm ) - PegSize / 2 )"
equation "d1884 = PegSize"
equation "d1885 = PegSize"
equation "d1886 = PegHeight"
equation "d1890 = ( BaseX + LeftRun + FaucetGap + RightRun - RightSideDepth ) + ( ( RightSideDepth ) - ( ( ( ( RightSideDepth ) - 11 mm ) - FootSize / 2 ) + ( FootSize ) ) )"
equation "d1891 = ( BaseY + Depth + ModuleGap ) + ( ( 11 mm ) - FootSize / 2 )"
equation "d1892 = FootSize"
equation "d1893 = FootSize"
equation "d1894 = FootHeight"
equation "d1896 = FootHeight"
equation "d1898 = ( BaseX + LeftRun + FaucetGap + RightRun - RightSideDepth ) + ( ( RightSideDepth ) - ( ( ( ( RightSideDepth ) - 11 mm ) - PegSize / 2 ) + ( PegSize ) ) )"
equation "d1899 = ( BaseY + Depth + ModuleGap ) + ( ( 11 mm ) - PegSize / 2 )"
equation "d1900 = PegSize"
equation "d1901 = PegSize"
equation "d1902 = PegHeight"
equation "d1906 = ( BaseX + LeftRun + FaucetGap + RightRun - RightSideDepth ) + ( ( RightSideDepth ) - ( ( ( 11 mm ) - FootSize / 2 ) + ( FootSize ) ) )"
equation "d1907 = ( BaseY + Depth + ModuleGap ) + ( ( ( RightReach ) - 11 mm ) - FootSize / 2 )"
equation "d1908 = FootSize"
equation "d1909 = FootSize"
equation "d1910 = FootHeight"
equation "d1912 = FootHeight"
equation "d1914 = ( BaseX + LeftRun + FaucetGap + RightRun - RightSideDepth ) + ( ( RightSideDepth ) - ( ( ( 11 mm ) - PegSize / 2 ) + ( PegSize ) ) )"
equation "d1915 = ( BaseY + Depth + ModuleGap ) + ( ( ( RightReach ) - 11 mm ) - PegSize / 2 )"
equation "d1916 = PegSize"
equation "d1917 = PegSize"
equation "d1918 = PegHeight"
equation "d1922 = ( BaseX + LeftRun + FaucetGap + RightRun - RightSideDepth ) + ( ( RightSideDepth ) - ( ( ( ( RightSideDepth ) - 11 mm ) - FootSize / 2 ) + ( FootSize ) ) )"
equation "d1923 = ( BaseY + Depth + ModuleGap ) + ( ( ( RightReach ) - 11 mm ) - FootSize / 2 )"
equation "d1924 = FootSize"
equation "d1925 = FootSize"
equation "d1926 = FootHeight"
equation "d1928 = FootHeight"
equation "d1930 = ( BaseX + LeftRun + FaucetGap + RightRun - RightSideDepth ) + ( ( RightSideDepth ) - ( ( ( ( RightSideDepth ) - 11 mm ) - PegSize / 2 ) + ( PegSize ) ) )"
equation "d1931 = ( BaseY + Depth + ModuleGap ) + ( ( ( RightReach ) - 11 mm ) - PegSize / 2 )"
equation "d1932 = PegSize"
equation "d1933 = PegSize"
equation "d1934 = PegHeight"
equation "d1936 = UpperDeckHeight - PanHeight"
equation "d1938 = ( BaseX ) + ( 0 mm )"
equation "d1939 = ( BaseY ) + ( 0 mm )"
equation "d1940 = TowerWidth"
equation "d1941 = Depth"
equation "d1942 = PanHeight"
equation "d1946 = ( BaseX ) + ( Wall )"
equation "d1948 = -( -( ( UpperDeckHeight - PanHeight ) + FloorMin + DrainExtension * tan(DrainSlope) + ( ( Depth ) - ( Wall ) ) * tan(DrainSlope) ) )"
equation "d1949 = ( ( BaseY ) + ( Wall ) )"
equation "d1950 = -( -( ( UpperDeckHeight - PanHeight ) + FloorMin + DrainExtension * tan(DrainSlope) + ( ( Depth ) - ( ( Depth ) - Wall ) ) * tan(DrainSlope) ) )"
equation "d1951 = ( ( BaseY ) + ( ( Depth ) - Wall ) )"
equation "d1952 = -( -( ( UpperDeckHeight - PanHeight ) + PanHeight + 1 mm ) )"
equation "d1953 = ( TowerWidth ) - 2 * Wall"
equation "d1955 = ( BaseX ) + ( ( TowerWidth - 35 mm ) - DrainWidth / 2 - Wall )"
equation "d1957 = -( -( UpperDeckHeight - PanHeight ) )"
equation "d1958 = ( ( BaseY ) + ( ( Depth ) - Wall ) )"
equation "d1959 = ( ( BaseY ) + ( ( Depth ) + DrainExtension ) )"
equation "d1960 = -( -( ( UpperDeckHeight - PanHeight ) + FloorMin + DrainExtension * tan(DrainSlope) + ( ( Depth ) - ( ( Depth ) + DrainExtension ) ) * tan(DrainSlope) ) )"
equation "d1961 = -( -( ( UpperDeckHeight - PanHeight ) + FloorMin + DrainExtension * tan(DrainSlope) + ( ( Depth ) - ( ( Depth ) - Wall ) ) * tan(DrainSlope) ) )"
equation "d1962 = DrainWidth + 2 * Wall"
equation "d1964 = ( BaseX ) + ( ( TowerWidth - 35 mm ) - DrainWidth / 2 - Wall )"
equation "d1966 = -( -( UpperDeckHeight - PanHeight ) )"
equation "d1967 = ( ( BaseY ) + ( ( Depth ) - Wall ) )"
equation "d1968 = ( ( BaseY ) + ( ( Depth ) + DrainExtension ) )"
equation "d1969 = -( -( ( ( UpperDeckHeight - PanHeight ) + FloorMin + DrainExtension * tan(DrainSlope) + ( ( Depth ) - ( ( Depth ) + DrainExtension ) ) * tan(DrainSlope) ) + ( 6 mm ) ) )"
equation "d1970 = -( -( ( ( UpperDeckHeight - PanHeight ) + FloorMin + DrainExtension * tan(DrainSlope) + ( ( Depth ) - ( ( Depth ) - Wall ) ) * tan(DrainSlope) ) + ( 6 mm ) ) )"
equation "d1971 = Wall"
equation "d1973 = ( BaseX ) + ( ( TowerWidth - 35 mm ) + DrainWidth / 2 )"
equation "d1975 = -( -( UpperDeckHeight - PanHeight ) )"
equation "d1976 = ( ( BaseY ) + ( ( Depth ) - Wall ) )"
equation "d1977 = ( ( BaseY ) + ( ( Depth ) + DrainExtension ) )"
equation "d1978 = -( -( ( ( UpperDeckHeight - PanHeight ) + FloorMin + DrainExtension * tan(DrainSlope) + ( ( Depth ) - ( ( Depth ) + DrainExtension ) ) * tan(DrainSlope) ) + ( 6 mm ) ) )"
equation "d1979 = -( -( ( ( UpperDeckHeight - PanHeight ) + FloorMin + DrainExtension * tan(DrainSlope) + ( ( Depth ) - ( ( Depth ) - Wall ) ) * tan(DrainSlope) ) + ( 6 mm ) ) )"
equation "d1980 = Wall"
equation "d1982 = ( BaseX ) + ( ( TowerWidth - 35 mm ) - DrainWidth / 2 )"
equation "d1984 = -( -( ( UpperDeckHeight - PanHeight ) + FloorMin + DrainExtension * tan(DrainSlope) + ( ( Depth ) - ( ( Depth ) - Wall ) ) * tan(DrainSlope) ) )"
equation "d1985 = ( ( BaseY ) + ( ( Depth ) - Wall ) )"
equation "d1986 = -( -( ( UpperDeckHeight - PanHeight ) + FloorMin + DrainExtension * tan(DrainSlope) + ( ( Depth ) - ( ( Depth ) + DrainExtension ) ) * tan(DrainSlope) ) )"
equation "d1987 = ( ( BaseY ) + ( ( Depth ) + DrainExtension ) )"
equation "d1988 = -( -( ( UpperDeckHeight - PanHeight ) + PanHeight + 1 mm ) )"
equation "d1989 = DrainWidth"
equation "d1991 = UpperDeckHeight - PanHeight"
equation "d1993 = ( BaseX ) + ( Wall )"
equation "d1994 = ( BaseY ) + ( Wall )"
equation "d1997 = PanHeight - DeckThick"
equation "d1999 = UpperDeckHeight - PanHeight"
equation "d2001 = ( BaseX ) + ( Wall )"
equation "d2002 = ( BaseY ) + ( ( Depth ) - Wall - 12 mm )"
equation "d2005 = PanHeight - DeckThick"
equation "d2007 = UpperDeckHeight - PanHeight"
equation "d2009 = ( BaseX ) + ( ( TowerWidth ) - Wall - 12 mm )"
equation "d2010 = ( BaseY ) + ( Wall )"
equation "d2013 = PanHeight - DeckThick"
equation "d2015 = UpperDeckHeight - PanHeight"
equation "d2017 = ( BaseX ) + ( ( TowerWidth ) - Wall - 12 mm )"
equation "d2018 = ( BaseY ) + ( ( Depth ) - Wall - 12 mm )"
equation "d2021 = PanHeight - DeckThick"
equation "d2023 = ( BaseX ) + ( ( TowerWidth - 35 mm ) - DrainWidth / 2 - Wall )"
equation "d2025 = -( -( ( UpperDeckHeight - PanHeight ) - ( 0.2 mm ) ) )"
equation "d2026 = ( ( BaseY ) + ( ( Depth ) + DrainExtension - 2 mm ) )"
equation "d2027 = ( ( BaseY ) + ( ( ( Depth ) + DrainExtension - 2 mm ) + ( 1 mm ) ) )"
equation "d2028 = -( -( ( UpperDeckHeight - PanHeight ) + ( 0.6 mm ) ) )"
equation "d2029 = DrainWidth + 2 * Wall"
equation "d2031 = ( UpperDeckHeight - PanHeight ) + PanHeight - DeckThick"
equation "d2033 = ( BaseX ) + ( Wall + DeckClearance )"
equation "d2034 = ( BaseY ) + ( Wall + DeckClearance )"
equation "d2035 = ( TowerWidth ) - 2 * ( Wall + DeckClearance )"
equation "d2036 = ( Depth ) - 2 * ( Wall + DeckClearance )"
equation "d2037 = DeckThick"
equation "d2039 = ( UpperDeckHeight - PanHeight ) + PanHeight - DeckThick"
equation "d2041 = ( BaseX ) + ( ( ( ( TowerWidth ) - ( 14 * SlotPitch + SlotWidth ) ) / 2 ) + ( 0 * SlotPitch ) )"
equation "d2042 = ( BaseY ) + ( Wall + DeckClearance + RimBorder )"
equation "d2043 = SlotWidth"
equation "d2044 = ( Depth ) - 2 * ( Wall + DeckClearance + RimBorder )"
equation "d2045 = DeckThick"
equation "d2047 = ( UpperDeckHeight - PanHeight ) + PanHeight - DeckThick"
equation "d2049 = ( BaseX ) + ( ( ( ( TowerWidth ) - ( 14 * SlotPitch + SlotWidth ) ) / 2 ) + ( 1 * SlotPitch ) )"
equation "d2050 = ( BaseY ) + ( Wall + DeckClearance + RimBorder )"
equation "d2051 = SlotWidth"
equation "d2052 = ( Depth ) - 2 * ( Wall + DeckClearance + RimBorder )"
equation "d2053 = DeckThick"
equation "d2055 = ( UpperDeckHeight - PanHeight ) + PanHeight - DeckThick"
equation "d2057 = ( BaseX ) + ( ( ( ( TowerWidth ) - ( 14 * SlotPitch + SlotWidth ) ) / 2 ) + ( 2 * SlotPitch ) )"
equation "d2058 = ( BaseY ) + ( Wall + DeckClearance + RimBorder )"
equation "d2059 = SlotWidth"
equation "d2060 = ( Depth ) - 2 * ( Wall + DeckClearance + RimBorder )"
equation "d2061 = DeckThick"
equation "d2063 = ( UpperDeckHeight - PanHeight ) + PanHeight - DeckThick"
equation "d2065 = ( BaseX ) + ( ( ( ( TowerWidth ) - ( 14 * SlotPitch + SlotWidth ) ) / 2 ) + ( 3 * SlotPitch ) )"
equation "d2066 = ( BaseY ) + ( Wall + DeckClearance + RimBorder )"
equation "d2067 = SlotWidth"
equation "d2068 = ( Depth ) - 2 * ( Wall + DeckClearance + RimBorder )"
equation "d2069 = DeckThick"
equation "d2071 = ( UpperDeckHeight - PanHeight ) + PanHeight - DeckThick"
equation "d2073 = ( BaseX ) + ( ( ( ( TowerWidth ) - ( 14 * SlotPitch + SlotWidth ) ) / 2 ) + ( 4 * SlotPitch ) )"
equation "d2074 = ( BaseY ) + ( Wall + DeckClearance + RimBorder )"
equation "d2075 = SlotWidth"
equation "d2076 = ( Depth ) - 2 * ( Wall + DeckClearance + RimBorder )"
equation "d2077 = DeckThick"
equation "d2079 = ( UpperDeckHeight - PanHeight ) + PanHeight - DeckThick"
equation "d2081 = ( BaseX ) + ( ( ( ( TowerWidth ) - ( 14 * SlotPitch + SlotWidth ) ) / 2 ) + ( 5 * SlotPitch ) )"
equation "d2082 = ( BaseY ) + ( Wall + DeckClearance + RimBorder )"
equation "d2083 = SlotWidth"
equation "d2084 = ( Depth ) - 2 * ( Wall + DeckClearance + RimBorder )"
equation "d2085 = DeckThick"
equation "d2087 = ( UpperDeckHeight - PanHeight ) + PanHeight - DeckThick"
equation "d2089 = ( BaseX ) + ( ( ( ( TowerWidth ) - ( 14 * SlotPitch + SlotWidth ) ) / 2 ) + ( 6 * SlotPitch ) )"
equation "d2090 = ( BaseY ) + ( Wall + DeckClearance + RimBorder )"
equation "d2091 = SlotWidth"
equation "d2092 = ( Depth ) - 2 * ( Wall + DeckClearance + RimBorder )"
equation "d2093 = DeckThick"
equation "d2095 = ( UpperDeckHeight - PanHeight ) + PanHeight - DeckThick"
equation "d2097 = ( BaseX ) + ( ( ( ( TowerWidth ) - ( 14 * SlotPitch + SlotWidth ) ) / 2 ) + ( 7 * SlotPitch ) )"
equation "d2098 = ( BaseY ) + ( Wall + DeckClearance + RimBorder )"
equation "d2099 = SlotWidth"
equation "d2100 = ( Depth ) - 2 * ( Wall + DeckClearance + RimBorder )"
equation "d2101 = DeckThick"
equation "d2103 = ( UpperDeckHeight - PanHeight ) + PanHeight - DeckThick"
equation "d2105 = ( BaseX ) + ( ( ( ( TowerWidth ) - ( 14 * SlotPitch + SlotWidth ) ) / 2 ) + ( 8 * SlotPitch ) )"
equation "d2106 = ( BaseY ) + ( Wall + DeckClearance + RimBorder )"
equation "d2107 = SlotWidth"
equation "d2108 = ( Depth ) - 2 * ( Wall + DeckClearance + RimBorder )"
equation "d2109 = DeckThick"
equation "d2111 = ( UpperDeckHeight - PanHeight ) + PanHeight - DeckThick"
equation "d2113 = ( BaseX ) + ( ( ( ( TowerWidth ) - ( 14 * SlotPitch + SlotWidth ) ) / 2 ) + ( 9 * SlotPitch ) )"
equation "d2114 = ( BaseY ) + ( Wall + DeckClearance + RimBorder )"
equation "d2115 = SlotWidth"
equation "d2116 = ( Depth ) - 2 * ( Wall + DeckClearance + RimBorder )"
equation "d2117 = DeckThick"
equation "d2119 = ( UpperDeckHeight - PanHeight ) + PanHeight - DeckThick"
equation "d2121 = ( BaseX ) + ( ( ( ( TowerWidth ) - ( 14 * SlotPitch + SlotWidth ) ) / 2 ) + ( 10 * SlotPitch ) )"
equation "d2122 = ( BaseY ) + ( Wall + DeckClearance + RimBorder )"
equation "d2123 = SlotWidth"
equation "d2124 = ( Depth ) - 2 * ( Wall + DeckClearance + RimBorder )"
equation "d2125 = DeckThick"
equation "d2127 = ( UpperDeckHeight - PanHeight ) + PanHeight - DeckThick"
equation "d2129 = ( BaseX ) + ( ( ( ( TowerWidth ) - ( 14 * SlotPitch + SlotWidth ) ) / 2 ) + ( 11 * SlotPitch ) )"
equation "d2130 = ( BaseY ) + ( Wall + DeckClearance + RimBorder )"
equation "d2131 = SlotWidth"
equation "d2132 = ( Depth ) - 2 * ( Wall + DeckClearance + RimBorder )"
equation "d2133 = DeckThick"
equation "d2135 = ( UpperDeckHeight - PanHeight ) + PanHeight - DeckThick"
equation "d2137 = ( BaseX ) + ( ( ( ( TowerWidth ) - ( 14 * SlotPitch + SlotWidth ) ) / 2 ) + ( 12 * SlotPitch ) )"
equation "d2138 = ( BaseY ) + ( Wall + DeckClearance + RimBorder )"
equation "d2139 = SlotWidth"
equation "d2140 = ( Depth ) - 2 * ( Wall + DeckClearance + RimBorder )"
equation "d2141 = DeckThick"
equation "d2143 = ( UpperDeckHeight - PanHeight ) + PanHeight - DeckThick"
equation "d2145 = ( BaseX ) + ( ( ( ( TowerWidth ) - ( 14 * SlotPitch + SlotWidth ) ) / 2 ) + ( 13 * SlotPitch ) )"
equation "d2146 = ( BaseY ) + ( Wall + DeckClearance + RimBorder )"
equation "d2147 = SlotWidth"
equation "d2148 = ( Depth ) - 2 * ( Wall + DeckClearance + RimBorder )"
equation "d2149 = DeckThick"
equation "d2151 = ( UpperDeckHeight - PanHeight ) + PanHeight - DeckThick"
equation "d2153 = ( BaseX ) + ( ( ( ( TowerWidth ) - ( 14 * SlotPitch + SlotWidth ) ) / 2 ) + ( 14 * SlotPitch ) )"
equation "d2154 = ( BaseY ) + ( Wall + DeckClearance + RimBorder )"
equation "d2155 = SlotWidth"
equation "d2156 = ( Depth ) - 2 * ( Wall + DeckClearance + RimBorder )"
equation "d2157 = DeckThick"
equation "d2159 = ( UpperDeckHeight - PanHeight ) + PanHeight - DeckThick"
equation "d2161 = ( BaseX ) + ( ( TowerWidth ) / 2 - 8 mm )"
equation "d2162 = ( BaseY ) + ( ( Depth ) - Wall - DeckClearance - 4 mm )"
equation "d2165 = DeckThick"
equation "d2169 = BaseX"
equation "d2170 = BaseY"
equation "d2171 = TowerFrame"
equation "d2172 = Depth"
equation "d2173 = UpperDeckHeight - PanHeight"
equation "d2175 = BaseX"
equation "d2177 = -( -( 8 mm ) )"
equation "d2178 = ( BaseY + 12 mm )"